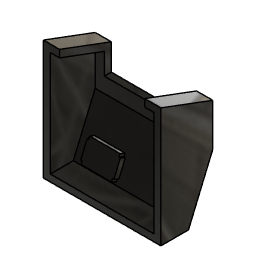
Back Part (Autodesk Fusion 360 design; units mm, degrees)
Autodesk Fusion 360 part; units mm, degrees
sketch "Sketch1" plane through (0, 0, 0) normal (1, 0, 0) x (0, 1, 0)
  line L0 (0, 0) -> (0, 1.433114)
  line L1 (0, 1.433114) -> (0, 86.433114)
  line L2 (0, 86.433114) -> (37.482031, 72.46539)
  line L3 (37.482031, 72.46539) -> (37.482031, 41.46539)
  line L4 (37.482031, 41.46539) -> (20, 0)
  line L5 (20, 0) -> (0, 0)
  dimension "d1" = 85
  dimension "d2" = 40
  dimension "d3" = 31
  dimension "d4" = 20
  dimension "d5" = 45
  constraint coincident L0.start L5.end
  constraint vertical L0
  constraint parallel L0 L1
  constraint parallel L1 L3
  constraint perpendicular L3 L5
  measures "d4" distance of L4.end L0.start
extrude "Extrude1" add sketch "Sketch1" along normal mid plane 85
sketch "Sketch2" plane through (0, 16.981517, -7.159499) normal (0, 0.921453, -0.38849) x (-1, 0, 0)
  line L0 (42.5, 52.769792) -> (-42.5, 52.769792)
  line L1 (-42.5, 52.769792) -> (-42.5, 7.769792)
  line L2 (-42.5, 7.769792) -> (42.5, 7.769792)
  line L3 (42.5, 7.769792) -> (42.5, 52.769792)
  circle A0 centre (20.020561, 38.010473) radius 4
  line L4 (25.020561, 33.010473) -> (15.020561, 33.010473)
  line L5 (15.020561, 33.010473) -> (15.020561, 43.010473)
  line L6 (15.020561, 43.010473) -> (25.020561, 43.010473)
  line L7 (25.020561, 43.010473) -> (25.020561, 33.010473)
  line L8 (25.020561, 33.010473) -> (15.020561, 43.010473) construction
  line L9 (15.020561, 33.010473) -> (25.020561, 43.010473) construction
  circle A1 centre (6.687228, 38.010473) radius 4
  line L10 (11.687228, 33.010473) -> (1.687228, 33.010473)
  line L11 (1.687228, 33.010473) -> (1.687228, 43.010473)
  line L12 (1.687228, 43.010473) -> (11.687228, 43.010473)
  line L13 (11.687228, 43.010473) -> (11.687228, 33.010473)
  circle A2 centre (-6.646105, 38.010473) radius 4
  line L14 (-1.646105, 33.010473) -> (-11.646105, 33.010473)
  line L15 (-11.646105, 33.010473) -> (-11.646105, 43.010473)
  line L16 (-11.646105, 43.010473) -> (-1.646105, 43.010473)
  line L17 (-1.646105, 43.010473) -> (-1.646105, 33.010473)
  circle A3 centre (-19.979439, 38.010473) radius 4
  line L18 (-14.979439, 33.010473) -> (-24.979439, 33.010473)
  line L19 (-24.979439, 33.010473) -> (-24.979439, 43.010473)
  line L20 (-24.979439, 43.010473) -> (-14.979439, 43.010473)
  line L21 (-14.979439, 43.010473) -> (-14.979439, 33.010473)
  circle A4 centre (-21, 21) radius 4
  circle A5 centre (-11, 21) radius 4
  line L22 (24, 18) -> (12, 18)
  line L23 (12, 18) -> (12, 24)
  line L24 (12, 24) -> (24, 24)
  line L25 (24, 24) -> (24, 18)
  line L26 (24, 18) -> (12, 24) construction
  line L27 (12, 18) -> (24, 24) construction
  line L28 (25.020561, 19.989762) -> (10.979439, 19.989762)
  line L29 (10.979439, 19.989762) -> (10.979439, 22.010238)
  line L30 (10.979439, 22.010238) -> (25.020561, 22.010238)
  line L31 (25.020561, 22.010238) -> (25.020561, 19.989762)
  line L32 (25.020561, 19.989762) -> (10.979439, 22.010238) construction
  line L33 (10.979439, 19.989762) -> (25.020561, 22.010238) construction
  point P0 (20.020561, 38.010473)
  point P1 (18, 21)
  point P2 (18, 21)
  dimension "d8" = 8
  dimension "d9" = 10
  dimension "d10" = 10
  dimension "d13" = -40
  dimension "d14" = 0
  dimension "d15" = 8
  dimension "d16" = 8
  constraint horizontal L4
  constraint perpendicular L4 L5
  constraint parallel L4 L6
  constraint parallel L5 L7
  constraint horizontal L22
  constraint perpendicular L22 L23
  constraint parallel L22 L24
  constraint parallel L23 L25
  constraint coincident L26 P2
  constraint coincident L27 P2
  constraint horizontal L28
  constraint perpendicular L28 L29
  constraint parallel L28 L30
  constraint parallel L29 L31
  constraint coincident L32 P2
  constraint coincident L33 P2
  constraint coincident P2 P1
  measures "d8" diameter of A0
  measures "d15" diameter of A4
  measures "d16" diameter of A5
extrude "Extrude2" add sketch "Sketch2" along normal blind 1 contours L4 L5 L6 L7 | L10 L11 L12 L13 | L14 L15 L16 L17 | L18 L19 L20 L21 picked at (19.920921, 33.347534) picked at (6.786868, 33.347534) picked at (-6.745746, 42.673411) picked at (-20.079079, 42.673411)
extrude "Extrude3" add sketch "Sketch2" along normal blind 4 contours A4 | A5 picked at (-19.854005, 20.054623) picked at (-11.296695, 22.299904)
extrude "Extrude4" cut sketch "Sketch2" against normal blind 4 contours L22 L23 L25 L28 | L23 L25 L28 L30 | L25 L28 L30 L31 | L23 L28 L29 L30 | L23 L24 L25 L30 picked at (20, 18.663254) picked at (20, 20.663254) picked at (24.340187, 21.336746) picked at (11.659813, 20.663254) picked at (20, 22.673492)
fillet "Fillet1" radius 4 2 edges at (24.72931, 28.263675, 9.304212) (14.72931, 28.263675, 9.304212)
shell "Shell1" thickness 5 removed faces 1 at (14.166667, 0, 57.622076)
sketch "Sketch3" plane through (0, 37.482031, 0) normal (0, 1, 0) x (-1, 0, 0)
  line L0 (42.5, 72.46539) -> (-42.5, 72.46539)
  line L1 (-42.5, 72.46539) -> (-42.5, 41.46539)
  line L2 (-42.5, 41.46539) -> (42.5, 41.46539)
  line L3 (42.5, 41.46539) -> (42.5, 72.46539)
  line L4 (30.816739, 53.426846) -> (-30.816739, 53.426846)
  line L5 (-30.816739, 53.426846) -> (-30.816739, 91.503934)
  line L6 (-30.816739, 91.503934) -> (30.816739, 91.503934)
  line L7 (30.816739, 91.503934) -> (30.816739, 53.426846)
  line L8 (30.816739, 53.426846) -> (-30.816739, 91.503934) construction
  line L9 (-30.816739, 53.426846) -> (30.816739, 91.503934) construction
  point P0 (0, 72.46539)
  constraint horizontal L4
  constraint perpendicular L4 L5
  constraint parallel L4 L6
  constraint parallel L5 L7
extrude "Extrude5" cut sketch "Sketch3" against normal blind 140 contours L0 L4 L5 L7 | L0 L5 L6 L7 picked at (-10.272246, 59.773027) picked at (-10.272246, 78.811572)
equation "d6 = ( 85 / 2 ) * 1 mm"
